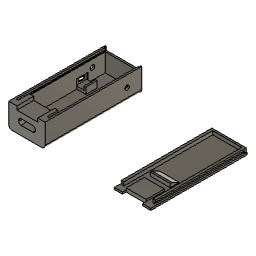
Coco_short_flat_Cover (Autodesk Fusion 360 design; units mm, degrees)
Autodesk Fusion 360 part; units mm, degrees
sketch "Skizze1" plane through (0, 0, 0) normal (0, 0, 1) x (1, 0, 0)
  line L0 (18, 20) -> (38, 20)
  line L1 (38, 20) -> (38, 73)
  line L2 (38, 73) -> (18, 73)
  line L3 (18, 73) -> (18, 20)
  line L4 (19, 23.2) -> (37, 23.2)
  line L5 (37, 23.2) -> (37, 72)
  line L6 (37, 72) -> (19, 72)
  line L7 (19, 72) -> (19, 23.2)
  line L8 (57, 90.4333) -> (57, 15.7858)
  line L9 (77, 72) -> (95, 72)
  line L10 (76, 73) -> (96, 73)
  line L11 (96, 73) -> (96, 20)
  line L12 (77, 23.2) -> (77, 72)
  line L13 (96, 20) -> (76, 20)
  line L14 (95, 72) -> (95, 23.2)
  line L15 (76, 20) -> (76, 73)
  line L16 (78, 71) -> (94, 71)
  line L17 (94, 71) -> (94, 23.2)
  line L18 (78, 23.2) -> (78, 71)
  line L19 (78, 71) -> (78, 73)
  line L20 (94, 71) -> (94, 73)
  line L21 (95, 72) -> (95, 73)
  line L22 (77, 72) -> (77, 73)
  line L23 (95, 23.2) -> (94, 23.2)
  line L24 (77, 23.2) -> (78, 23.2)
  line L25 (-15, -7.8) -> (-15, -6.8)
  line L26 (-15, -6.8) -> (-13, -6.8)
  line L27 (-13, -6.8) -> (-13, -15)
  line L28 (-13, -15) -> (-15, -15)
  line L29 (-15, -15) -> (-15, -14)
  line L30 (-15, -14) -> (-13.6, -14)
  line L31 (-13.6, -14) -> (-13.6, -7.8)
  line L32 (-13.6, -7.8) -> (-15, -7.8)
  dimension "d3" = 53
  dimension "d4" = 20
  dimension "d5" = 1
  dimension "d6" = 1
  dimension "d7" = 19
  dimension "d8" = 49.8
  dimension "d13" = 1
  dimension "d15" = 1
  dimension "d16" = 17
  dimension "d71" = 38
  dimension "d72" = 73
  dimension "d212" = 15
  dimension "d213" = 15
  dimension "d214" = 1
  dimension "d215" = 2
  dimension "d216" = 1.4
  dimension "d217" = 7.2
  dimension "d218" = 8.2
  dimension "d246" = 114
  constraint horizontal L0
  constraint vertical L1
  constraint horizontal L2
  constraint vertical L3
  constraint horizontal L4
  constraint vertical L5
  constraint horizontal L6
  constraint vertical L7
  constraint vertical L8
  constraint symmetric L0.start L8 L11.end
  constraint symmetric L0.end L8 L13.end
  constraint symmetric L1.end L8 L10.start
  constraint symmetric L2.end L8 L10.end
  constraint symmetric L4.start L8 L14.end
  constraint symmetric L4.end L8 L12.start
  constraint symmetric L5.end L8 L9.start
  constraint symmetric L6.end L8 L9.end
  constraint horizontal L16
  constraint vertical L17
  constraint vertical L18
  constraint coincident L10 L19.end
  constraint perpendicular L10 L19
  constraint coincident L10 L20.end
  constraint perpendicular L10 L20
  constraint coincident L10 L21.end
  constraint perpendicular L10 L21
  constraint coincident L10 L22.end
  constraint perpendicular L10 L22
  constraint perpendicular L14 L23
  constraint perpendicular L12 L24
  constraint vertical L25
  constraint perpendicular L25 L26
  constraint perpendicular L26 L27
  constraint perpendicular L27 L28
  constraint perpendicular L28 L29
  constraint perpendicular L27 L30
  constraint perpendicular L30 L31
  constraint perpendicular L25 L32
  constraint collinear L25 L29
  measures "d3" distance of L0 L2
  measures "d4" distance of L1 L3
  measures "d5" distance of L2 L6
  measures "d6" distance of L1 L5
  measures "d7" distance of L1 L7
  measures "d8" distance of L2 L4
  measures "d13" distance of L9 L16
  measures "d15" distance of L14 L17
  measures "d16" distance of L14 L18
  measures "d71" distance of origin L1
  measures "d72" distance of origin L2
  measures "d212" distance of origin L28
  measures "d213" distance of origin L29
  measures "d214" distance of L28 L30
  measures "d215" distance of L27 L29
  measures "d216" distance of L29 L31
  measures "d217" distance of L28 L32
  measures "d218" distance of L26 L28
extrude "Extrusion1" add sketch "Skizze1" along normal blind 13 contours L0 L1 L2 L3 makes body 1
extrude "Extrusion2" add sketch "Skizze1" along normal blind 1 contours L4 L5 L6 L7 bodies 1
extrude "Extrusion3" add sketch "Skizze1" along normal blind 3 separate body contours L9 L10 L19 L22 | L9 L12 L18 L19 L24 | L9 L10 L19 L20 | L9 L10 L20 L21 | L9 L14 L17 L20 L23 makes body 2
extrude "Extrusion4" add sketch "Skizze1" along normal blind 1 contours L9 L10 L19 L22 | L10 L11 L12 L13 L14 L15 L16 L17 L18 L21 L22 L23 L24 | L9 L10 L19 L20 | L9 L16 L19 L20 | L9 L10 L20 L21 bodies 2
fillet "Abrundung1" radius 2 2 edges at (38, 46.5, 0) (18, 46.5, 0) on bodies 1
ref_plane "Arbeitsebene1" through (28, 0, 0) normal (1, 0, 0) x (0, 1, 0)
sketch "Skizze2" plane through (28, 0, 0) normal (1, 0, 0) x (0, 1, 0)
  line L0 (23.2, 12) -> (73, 12)
  line L1 (73, 12) -> (73, 11)
  line L2 (73, 11) -> (23.2, 11)
  line L3 (23.2, 11) -> (23.2, 12)
  dimension "d25" = 11
  dimension "d26" = 49.8
  dimension "d27" = 1
  dimension "d44" = 73
  constraint horizontal L0
  constraint vertical L1
  constraint horizontal L2
  constraint vertical L3
  measures "d25" vertical distance of origin L2.end
  measures "d26" distance of L1 L3
  measures "d27" distance of L0 L2
  measures "d44" distance of origin L1
extrude "Extrusion10" cut sketch "Skizze2" along normal mid plane 19 bodies 1
sketch "Skizze3" plane through (0, 20, 0) normal (0, -1, 0) x (1, 0, 0)
  arc A0 (18, 2) -> (20, 0) centre (20, 2) ccw
  arc A1 (36, 0) -> (38, 2) centre (36, 2) ccw
  line L0 (38, 2) -> (38, 13)
  line L1 (38, 13) -> (18, 13)
  line L2 (18, 13) -> (18, 2)
  line L3 (24.69, 4.89) -> (31.31, 4.89)
  line L4 (24.69, 8.11) -> (31.31, 8.11)
  line L5 (28, 12.5188) -> (28, 0.4317)
  arc A2 (23.49, 6.09) -> (24.69, 4.89) centre (24.69, 6.09) ccw
  line L6 (23.49, 6.09) -> (23.49, 6.91)
  arc A3 (24.69, 8.11) -> (23.49, 6.91) centre (24.69, 6.91) ccw
  arc A4 (32.51, 6.91) -> (31.31, 8.11) centre (31.31, 6.91) ccw
  arc A5 (31.31, 4.89) -> (32.51, 6.09) centre (31.31, 6.09) ccw
  line L7 (32.51, 6.91) -> (32.51, 6.09)
  line L8 (22.5, 13) -> (34, 13)
  line L9 (34, 13) -> (34, 11)
  line L10 (34, 11) -> (22.5, 11)
  line L11 (22.5, 11) -> (22.5, 13)
  line L12 (20, 0) -> (36, 0)
  dimension "d30" = 6.62
  dimension "d32" = 6.62
  dimension "d34" = 3.31
  dimension "d35" = 3.31
  dimension "d36" = 1.2
  dimension "d37" = 1.2
  dimension "d171" = 2
  dimension "d204" = 6
  dimension "d205" = 11.5
  dimension "d269" = 4.89
  dimension "d270" = 8.11
  constraint horizontal L3
  constraint horizontal L4
  constraint tangent L3 A2
  constraint vertical L6
  constraint tangent L6 A3
  constraint tangent L4 A3
  constraint tangent A2 L6
  constraint tangent L4 A4
  constraint tangent L3 A5
  constraint perpendicular L1 L7
  constraint tangent A5 L7
  constraint tangent A4 L7
  constraint horizontal L8
  constraint vertical L9
  constraint horizontal L10
  constraint vertical L11
  constraint coincident L1 L8.start
  measures "d30" distance of L3.start L3.end
  measures "d32" distance of L4.start L4.end
  measures "d34" distance of L3.end L5
  measures "d35" distance of L4.end L5
  measures "d36" radius of A3
  measures "d37" radius of A4
  measures "d171" distance of L8 L10
  measures "d204" distance of L5 L9
  measures "d205" distance of L9 L11
  measures "d269" distance of origin L3
  measures "d270" distance of origin L4
extrude "Extrusion6" cut sketch "Skizze3" against normal blind 3.2 contours L1 L8 L9 L10 L11 | L3 L4 L5 A2 L6 A3 | L3 L4 L5 A4 A5 L7 bodies 1
fillet "Abrundung2" [suppressed]
sketch "Skizze7" plane through (0, 73, 0) normal (0, 1, 0) x (-1, 0, 0)
  arc A0 (-20, 0) -> (-18, 2) centre (-20, 2) ccw
  line L0 (-18, 2) -> (-18, 13)
  line L1 (-38, 13) -> (-38, 2)
  arc A1 (-38, 2) -> (-36, 0) centre (-36, 2) ccw
  line L2 (-36, 0) -> (-20, 0)
  line L3 (-37.5, 13) -> (-18.5, 13)
  line L4 (-18.5, 13) -> (-18.5, 12)
  line L5 (-18.5, 12) -> (-37.5, 12)
  line L6 (-37.5, 12) -> (-37.5, 13)
  line L7 (-28, 12.5188) -> (-28, 0.4317)
  circle A2 centre (-31.5, 6) radius 1.25
  line L8 (-18, 13) -> (-38, 13)
  line L9 (-18.5, 12) -> (-18.5, 11)
  line L10 (-18.5, 11) -> (-37.5, 11)
  line L11 (-37.5, 11) -> (-37.5, 12)
  line L12 (-37.5, 12) -> (-18.5, 12)
  dimension "d59" = 19
  dimension "d60" = 9.5
  dimension "d116" = 2.5
  dimension "d117" = 6
  dimension "d206" = 3.5
  dimension "d264" = 13
  dimension "d265" = 1
  constraint horizontal L3
  constraint vertical L4
  constraint horizontal L5
  constraint vertical L6
  measures "d59" distance of L4 L6
  measures "d60" distance of L4 L7
  measures "d116" diameter of A2
  measures "d117" distance of L2 A2.centre
  measures "d206" distance of L7 A2.centre
  measures "d264" distance of origin L3
  measures "d265" distance of L3 L5
extrude "Extrusion11" cut sketch "Skizze7" against normal blind 1 contours L3 L4 L5 L6 L8 L12 bodies 1
sketch "Skizze8" plane through (95, 0, 0) normal (1, 0, 0) x (0, 1, 0)
  line L0 (23.2, 1) -> (73, 1)
  line L1 (73, 1) -> (73, 3)
  line L2 (73, 3) -> (23.2, 3)
  line L3 (23.2, 3) -> (73, 3)
  line L4 (72, 2.1) -> (23.2, 2.1)
  line L5 (23.2, 2.1) -> (23.2, 3)
  line L6 (73, 3) -> (73, 1)
  line L7 (72, 1) -> (72, 2.1)
  line L8 (23.2, 3) -> (23.2, 1)
  dimension "d63" = 0.9
  dimension "d125" = 1
  constraint horizontal L3
  constraint horizontal L4
  constraint vertical L5
  constraint coincident L2.end L3.start
  constraint coincident L0.end L1.start
  constraint coincident L0 L7.start
  constraint coincident L4 L7.end
  constraint perpendicular L4 L7
  constraint coincident L1.end L2.start
  measures "d63" distance of L2.end L4.end
  measures "d125" distance of L6 L7
extrude "Extrusion12" add sketch "Skizze8" along normal blind 0.4 contours L0 L1 L2 L3 L4 L5 L6 L7 L8 bodies 2
sketch "Skizze9" plane through (77, 0, 0) normal (-1, 0, 0) x (0, -1, 0)
  line L0 (-23.2, 3) -> (-23.2, 2.1)
  line L1 (-23.2, 2.1) -> (-72, 2.1)
  line L2 (-73, 1) -> (-73, 3)
  line L3 (-73, 1) -> (-72, 1)
  line L4 (-72, 2.1) -> (-72, 1)
  line L5 (-23.2, 1) -> (-23.2, 3)
  line L6 (-73, 1) -> (-23.2, 1)
  line L7 (-73, 3) -> (-23.2, 3)
  line L8 (-73, 1) -> (-73, 3)
  line L9 (-23.2, 1) -> (-23.2, 3)
  dimension "d127" = 1
  dimension "d268" = 0.9
  constraint vertical L0
  constraint horizontal L1
  constraint vertical L2
  constraint coincident L1 L4.start
  constraint coincident L1.end L4
  constraint coincident L0.start L5.end
  constraint collinear L2 L8
  constraint collinear L3 L6
  measures "d127" distance of L2 L4
  measures "d268" distance of L1 L7
extrude "Extrusion13" add sketch "Skizze9" along normal blind 0.4 contours L0 L1 L2 L3 L4 L5 L6 L7 L8 L9 bodies 2
sketch "Skizze10" plane through (0, 0, 1) normal (0, 0, 1) x (-1, 0, 0)
  line L0 (-76, -20) -> (-96, -20)
  line L1 (-94, -23.2) -> (-94, -72)
  line L2 (-80.5, -32) -> (-91.5, -32)
  line L3 (-80.5, -32) -> (-80.5, -22)
  line L4 (-80.5, -22) -> (-91.5, -22)
  line L5 (-91.5, -22) -> (-91.5, -32)
  line L6 (-80.5, -40.2) -> (-91.5, -40.2)
  line L7 (-91.5, -40.2) -> (-91.5, -35.2)
  line L8 (-91.5, -35.2) -> (-80.5, -35.2)
  line L9 (-80.5, -35.2) -> (-80.5, -40.2)
  line L10 (-95.4, -72) -> (-95, -72)
  line L11 (-95, -72) -> (-95, -23.2)
  line L12 (-95, -23.2) -> (-94, -23.2)
  line L13 (-76.6, -73) -> (-76, -73)
  line L14 (-76, -73) -> (-76, -20)
  line L15 (-96, -20) -> (-96, -73)
  line L16 (-96, -73) -> (-95.4, -73)
  line L17 (-95.4, -73) -> (-95.4, -72)
  line L18 (-76.6, -72) -> (-76.6, -73)
  line L19 (-76.6, -73) -> (-95.4, -73)
  line L20 (-94, -72) -> (-78, -72)
  line L21 (-78, -72) -> (-78, -23.2)
  line L22 (-78, -23.2) -> (-77, -23.2)
  line L23 (-77, -23.2) -> (-77, -72)
  dimension "d226" = 2
  dimension "d227" = 12
  dimension "d249" = 20.2
  dimension "d250" = 15.2
  dimension "d271" = 15.5
  dimension "d272" = 4.5
  constraint perpendicular L2 L3
  constraint perpendicular L2 L5
  constraint horizontal L6
  constraint vertical L7
  constraint horizontal L8
  constraint vertical L9
  constraint collinear L3 L9
  constraint collinear L5 L7
  measures "d226" distance of L0 L4
  measures "d227" distance of L0 L2
  measures "d249" distance of L0 L6
  measures "d250" distance of L0 L8
  measures "d271" distance of L5 L14
  measures "d272" distance of L3 L14
extrude "Extrusion30" add sketch "Skizze10" along normal blind 1 contours L2 L3 L4 L5 bodies 2
extrude "Extrusion33" add sketch "Skizze10" along normal blind 2 contours L6 L7 L8 L9 bodies 2
chamfer "Fase2" distance 4 distance2 2 1 edges at (86, 40.2, 3) measured on face at (84.1667, 38.5333, 3) on bodies 2
sketch "Skizze11" plane through (18, 0, 0) normal (-1, 0, 0) x (0, -1, 0)
  line L0 (-73, 2) -> (-20, 2)
  line L1 (-20, 2) -> (-20, 13)
  line L2 (-20, 13) -> (-73, 13)
  line L3 (-73, 13) -> (-73, 2)
  line L4 (-61.2, 3.4) -> (-57.9, 3.4)
  line L5 (-57.9, 3.4) -> (-57.9, 5)
  line L6 (-57.9, 5) -> (-61.2, 5)
  line L7 (-61.2, 5) -> (-61.2, 3.4)
  line L8 (-56.5, 5.95) -> (-56.5, 2.45)
  line L9 (-56.5, 5.95) -> (-62.6, 5.95)
  line L10 (-62.6, 5.95) -> (-62.6, 2.45)
  line L11 (-62.6, 2.45) -> (-56.5, 2.45)
  circle A0 centre (-65, 7) radius 1.25
  dimension "d76" = 3.3
  dimension "d77" = 1.6
  dimension "d78" = 15.1
  dimension "d179" = 3.95
  dimension "d180" = 3.5
  dimension "d181" = 16.5
  dimension "d182" = 6.1
  dimension "d193" = 3
  dimension "d258" = 6
  dimension "d259" = 8
  dimension "d260" = 2.5
  constraint horizontal L4
  constraint vertical L5
  constraint horizontal L6
  constraint vertical L7
  constraint perpendicular L6 L8
  constraint perpendicular L8 L9
  constraint perpendicular L0 L10
  constraint horizontal L11
  measures "d76" distance of L4.start L4.end
  measures "d77" distance of L4.start L6.end
  measures "d78" distance of L3 L5
  measures "d179" distance of L0 L9
  measures "d180" distance of L9 L11
  measures "d181" distance of L3 L8
  measures "d182" distance of L8 L10
  measures "d193" distance of L0 L6
  measures "d258" distance of L2 A0.centre
  measures "d259" distance of L3 A0.centre
  measures "d260" diameter of A0
extrude "Extrusion15" cut sketch "Skizze11" against normal blind 1 contours L4 L5 L6 L7 bodies 1
extrude "Extrusion34" cut sketch "Skizze11" against normal blind 20 contours A0 bodies 1
sketch "Skizze12" plane through (0, 0, 1) normal (0, 0, 1) x (-1, 0, 0)
  line L0 (-19, -72) -> (-19, -23.2)
  line L1 (-37, -23.2) -> (-37, -72)
  line L2 (-23, -62.5) -> (-23, -56.4)
  line L3 (-24, -62.5) -> (-24, -56.4)
  line L4 (-24, -56.4) -> (-23, -56.4)
  line L5 (-24, -62.5) -> (-23, -62.5)
  line L6 (-18, -73) -> (-18, -20)
  line L7 (-23, -62.5) -> (-19, -62.5)
  line L8 (-23, -56.4) -> (-19, -56.4)
  line L9 (-18.5, -73) -> (-18, -73)
  line L10 (-19, -23.2) -> (-37, -23.2)
  line L11 (-34, -20) -> (-38, -20)
  line L12 (-18, -20) -> (-22.5, -20)
  dimension "d177" = 6
  dimension "d178" = 5
  dimension "d253" = 10.5
  dimension "d254" = 16.6
  constraint vertical L2
  constraint perpendicular L3 L4
  constraint vertical L3
  constraint perpendicular L2 L5
  constraint coincident L0 L7.end
  constraint perpendicular L0 L7
  constraint coincident L0 L8.end
  constraint perpendicular L0 L8
  measures "d177" distance of L3 L6
  measures "d178" distance of L2 L6
  measures "d253" distance of L7 L9
  measures "d254" distance of L8 L9
extrude "Extrusion17" add sketch "Skizze12" along normal blind 3.5 contours L2 L3 L4 L5 bodies 1
extrude "Extrusion27" add sketch "Skizze12" along normal blind 1.45 contours L0 L2 L7 L8 bodies 1
sketch "Skizze13" plane through (19, 0, 0) normal (1, 0, 0) x (0, 1, 0)
  line L0 (72, 1) -> (72, 11)
  line L1 (62.5, 1) -> (72, 1)
  line L2 (61.2, 3.4) -> (57.9, 3.4)
  line L3 (57.9, 3.4) -> (57.9, 5)
  line L4 (57.9, 5) -> (61.2, 5)
  line L5 (61.2, 5) -> (61.2, 3.4)
  line L6 (-70.5, 1.05) -> (-64.4, 1.05)
  line L7 (-64.4, 4.55) -> (-64.4, 1.05)
  line L8 (-65.9, 2) -> (-65.9, 3.6)
  line L9 (-69, 2) -> (-65.9, 2)
  line L10 (-64.4, 4.55) -> (-70.5, 4.55)
  line L11 (-70.5, 4.55) -> (-70.5, 1.05)
  line L12 (-69, 3.6) -> (-69, 2)
  line L13 (-65.9, 3.6) -> (-69, 3.6)
  line L14 (56.4, 5.95) -> (56.4, 1)
  line L15 (62.5, 1) -> (62.5, 5.95)
  line L16 (62.5, 5.95) -> (56.4, 5.95)
  line L17 (73, 13) -> (73, 2)
  line L18 (62.6, 2.45) -> (56.5, 2.45)
  line L19 (62.5, 2.45) -> (62.5, 1)
  line L20 (56.4, 1) -> (56.4, 2.45)
  line L21 (56.4, 2.45) -> (62.5, 2.45)
  circle A0 centre (65, 7) radius 1.25
  line L22 (23.2, 11) -> (23.2, 1)
  line L23 (72, 11) -> (23.2, 11)
  line L24 (23.2, 1) -> (56.4, 1)
  point P0 (-83, 2)
  dimension "d183" = 3.1
  dimension "d184" = 1.6
  dimension "d185" = 3.5
  dimension "d186" = 6.1
  dimension "d187" = 6.1
  dimension "d188" = 16.6
  dimension "d189" = 3.5
  constraint horizontal L9
  constraint vertical L8
  constraint horizontal L13
  constraint vertical L12
  constraint perpendicular L7 L13
  constraint perpendicular L7 L10
  constraint horizontal L6
  constraint coincident L1 L14.end
  constraint perpendicular L1 L14
  constraint coincident L1 L15.start
  constraint perpendicular L1 L15
  constraint perpendicular L14 L16
  measures "d183" distance of L9.start L8.start
  measures "d184" distance of L9.start L12.start
  measures "d185" distance of L6 L10
  measures "d186" distance of L7 L11
  measures "d187" distance of L14 L15
  measures "d188" distance of L14 L17
  measures "d189" distance of L16 L18
extrude "Extrusion26" cut sketch "Skizze13" against normal blind 0.5 contours L14 L15 L16 L18 L21 bodies 1
sketch "Skizze14" plane through (0, 20, 0) normal (0, -1, 0) x (1, 0, 0)
  line L0 (76, 0) -> (96, 0)
  line L1 (80.5, 1) -> (91.5, 1)
  line L2 (91.5, 1) -> (91.5, 0)
  line L3 (91.5, 0) -> (80.5, 0)
  line L4 (80.5, 0) -> (80.5, 1)
  line L5 (96, 0) -> (96, 1)
  line L6 (76, 1) -> (76, 0)
  line L7 (96, 1) -> (76, 1)
  dimension "d106" = 11
  dimension "d267" = 15.5
  constraint horizontal L1
  constraint vertical L2
  constraint horizontal L3
  constraint vertical L4
  constraint collinear L0 L3
  constraint collinear L1 L7
  measures "d106" distance of L2 L4
  measures "d267" distance of L2 L6
extrude "Extrusion20" cut sketch "Skizze14" against normal blind 2 contours L0 L1 L2 L3 L4 L7 bodies 2
ref_plane "Arbeitsebene2" through (0, 0, 6) normal (0, 0, 1) x (1, 0, 0)
sketch "Skizze15" plane through (0, 0, 6) normal (0, 0, 1) x (1, 0, 0)
  line L0 (24, 73) -> (24, 76)
  arc A0 (27, 79) -> (24, 76) centre (27, 76) ccw
  arc A1 (34, 76) -> (31, 79) centre (31, 76) ccw
  line L1 (27, 79) -> (31, 79)
  line L2 (34, 76) -> (34, 73)
  line L3 (18, 73) -> (18, 20)
  line L4 (18.5, 73) -> (18, 73)
  dimension "d112" = 16
  dimension "d113" = 10
  dimension "d114" = 3
  dimension "d115" = 3
  dimension "d255" = 3
  constraint vertical L0
  constraint tangent L0 A0
  constraint tangent A0 L1
  constraint perpendicular L1 L2
  constraint tangent A1 L1
  constraint tangent A1 L2
  constraint vertical L2
  measures "d112" distance of L2 L3
  measures "d113" distance of L0 L2
  measures "d114" radius of A0
  measures "d115" radius of A1
  measures "d255" distance of A0.centre L4
sweep "Sweeping1" [suppressed]
fillet "Abrundung5" [suppressed]
sketch "Skizze16" plane through (0, 0, 0) normal (0, 0, -1) x (1, 0, 0)
  line L0 (20, -20) -> (20, -73)
  line L1 (20, -73) -> (36, -73)
  line L2 (36, -73) -> (36, -20)
  circle A0 centre (28, -28) radius 7
  circle A1 centre (28, -28) radius 6
  line L3 (38, -73) -> (38, -20)
  circle A2 centre (28, -28) radius 3
  circle A3 centre (28, -28) radius 1.5
  line L4 (22.9049, -23.2) -> (33.0951, -23.2)
  line L5 (36, -20) -> (20, -20)
  dimension "d128" = 14
  dimension "d130" = 10
  dimension "d131" = 1
  dimension "d132" = 6
  dimension "d133" = 3
  dimension "d273" = 8
  dimension "d274" = 3.2
  constraint concentric A0 A1
  constraint concentric A0 A2
  constraint concentric A1 A3
  constraint coincident A0 L4.start
  constraint coincident A0 L4.end
  constraint horizontal L4
  measures "d128" diameter of A0
  measures "d130" distance of A0.centre L3
  measures "d131" distance of A0 A1
  measures "d132" diameter of A2
  measures "d133" diameter of A3
  measures "d273" distance of A0.centre L5
  measures "d274" distance of L4 L5
extrude "Extrusion32" cut sketch "Skizze16" against normal blind 1 contours A0 A1 L4 | A2 | A3 picked at (23.4498, -32.8545) bodies 1
extrude "Extrusion22" add sketch "Skizze16" against normal blind 1 separate body contours A0 A1 L4 | A2 | A3 picked at (23.4498, -32.8545) makes body 3 at (27.9253, 27.1355, 0) makes body 4 at (25.6704, 34.601, 0.6667)
sketch "Skizze17" plane through (0, 23.2, 0) normal (0, 1, 0) x (-1, 0, 0)
  line L0 (-20.1, 13) -> (-20.1, 12)
  line L1 (-35.9, 12) -> (-35.9, 13)
  line L2 (-37, 12) -> (-37, 13)
  line L3 (-34, 13) -> (-37, 13)
  line L4 (-38, 2) -> (-38, 13)
  line L5 (-34, 11) -> (-22.5, 11)
  line L6 (-35, 10) -> (-35, 12)
  line L7 (-35.9, 12) -> (-35, 12)
  line L8 (-21.5, 12) -> (-20.1, 12)
  line L9 (-20.1, 13) -> (-22.5, 13)
  line L10 (-21.5, 12) -> (-21.5, 10)
  line L11 (-35.9, 13) -> (-34, 13)
  line L12 (-37, 12) -> (-37.5, 12)
  line L13 (-35, 10) -> (-21.5, 10)
  line L14 (-22.5, 11) -> (-22.5, 13)
  line L15 (-22.5, 13) -> (-22.5, 11)
  line L16 (-34, 11) -> (-34, 13)
  line L17 (-37, 13) -> (-37, 12)
  line L18 (-19, 1) -> (-19, 11)
  line L19 (-34, 13) -> (-34, 11)
  line L20 (-37.5, 12) -> (-37.5, 11)
  line L21 (-37.5, 11) -> (-37, 11)
  line L22 (-37, 11) -> (-37, 1)
  line L23 (-37, 1) -> (-33.0951, 1)
  line L24 (-33.0951, 1) -> (-33.0951, 0)
  line L25 (-33.0951, 0) -> (-31.6, 0)
  line L26 (-31.6, 0) -> (-31.6, 1)
  line L27 (-31.6, 1) -> (-24.4, 1)
  line L28 (-24.4, 1) -> (-24.4, 0)
  line L29 (-24.4, 0) -> (-22.9049, 0)
  line L30 (-22.9049, 0) -> (-22.9049, 1)
  line L31 (-22.9049, 1) -> (-19, 1)
  line L32 (-19, 11) -> (-18.5, 11)
  line L33 (-18.5, 11) -> (-18.5, 12)
  line L34 (-18.5, 12) -> (-19, 12)
  line L35 (-19, 12) -> (-19, 13)
  line L36 (-19, 13) -> (-22.5, 13)
  line L37 (-23.49, 6.91) -> (-23.49, 6.09)
  arc A0 (-24.69, 4.89) -> (-23.49, 6.09) centre (-24.69, 6.09) ccw
  line L38 (-24.69, 4.89) -> (-31.31, 4.89)
  arc A1 (-32.51, 6.09) -> (-31.31, 4.89) centre (-31.31, 6.09) ccw
  line L39 (-32.51, 6.09) -> (-32.51, 6.91)
  arc A2 (-31.31, 8.11) -> (-32.51, 6.91) centre (-31.31, 6.91) ccw
  line L40 (-31.31, 8.11) -> (-24.69, 8.11)
  arc A3 (-23.49, 6.91) -> (-24.69, 8.11) centre (-24.69, 6.91) ccw
  line L41 (-18.5, 12) -> (-19, 12)
  line L42 (-37, 12) -> (-37.5, 12)
  line L43 (-37, 13) -> (-34, 13)
  dimension "d174" = 2.1
  dimension "d175" = 17.9
  dimension "d266" = 1
  dimension "d275" = 3
  dimension "d277" = 1
  dimension "d278" = 2
  dimension "d279" = 1
  constraint vertical L0
  constraint vertical L1
  constraint perpendicular L6 L7
  constraint vertical L6
  constraint perpendicular L0 L8
  constraint coincident L3.start L11.end
  constraint collinear L7 L8
  constraint perpendicular L10 L13
  constraint perpendicular L9 L14
  constraint collinear L14 L15
  constraint horizontal L5
  constraint vertical L19
  measures "d174" distance of L1 L4
  measures "d175" distance of L0 L4
  measures "d266" distance of L7 L11
  measures "d275" distance of L11 L13
  measures "d277" distance of L6 L16
  measures "d278" distance of L5 L11
  measures "d279" distance of L10 L14
extrude "Extrusion25" add sketch "Skizze17" along normal blind 6 contours L0 L1 L3 L5 L6 L7 L8 L9 L10 L11 L13 L14 L15 L16 L19 L36 L43 bodies 1
extrude "Extrusion28" add sketch "Skizze1" along normal blind 4 separate body contours L25 L26 L27 L28 L29 L30 L31 L32 makes body 5
sketch "Skizze18" plane through (-13.6, 0, 0) normal (-1, 0, 0) x (0, -1, 0)
  line L0 (7.8, 0) -> (14, 0)
  line L1 (14, 0) -> (14, 4)
  line L2 (14, 4) -> (7.8, 4)
  line L3 (7.8, 4) -> (7.8, 0)
  line L4 (7.8, 0) -> (14, 0)
  line L5 (14, 0) -> (14, 1.5)
  line L6 (14, 1.5) -> (7.8, 1.5)
  line L7 (7.8, 1.5) -> (7.8, 0)
  dimension "d221" = 1.5
  constraint horizontal L4
  constraint vertical L5
  constraint horizontal L6
  constraint vertical L7
  constraint coincident L1 L5.end
  constraint coincident L0.start L3.end
  measures "d221" distance of L4 L6
extrude "Extrusion29" cut sketch "Skizze18" against normal blind 0.6 contours L0 L1 L3 L4 L5 L6 L7 bodies 5
sketch "Skizze19" plane through (0, 0, 6) normal (0, 0, 1) x (1, 0, 0)
  circle A0 centre (29, 80) radius 10
  line L0 (18, 73) -> (18, 20)
  line L1 (14, 95) -> (44, 95)
  line L2 (44, 95) -> (44, 73)
  line L3 (14, 73) -> (14, 95)
  line L4 (18.5, 73) -> (18, 73)
  line L5 (44, 73) -> (14, 73)
  dimension "d231" = 20
  dimension "d233" = 11
  dimension "d234" = 15
  dimension "d235" = 30
  dimension "d236" = 15
  dimension "d256" = 7
  dimension "d257" = 7
  constraint horizontal L1
  constraint vertical L2
  constraint vertical L3
  constraint perpendicular L3 L5
  measures "d231" diameter of A0
  measures "d233" distance of A0.centre L0
  measures "d234" distance of A0.centre L2
  measures "d235" distance of L2 L3
  measures "d236" distance of A0.centre L1
  measures "d256" distance of A0.centre L4
  measures "d257" distance of A0.centre L5
hidden bodies 3 4 5
equation "d3 = Länge + Wandstärke"
equation "d4 = Breite + 2 * Wandstärke"
equation "d5 = Wandstärke"
equation "d6 = Wandstärke"
equation "d7 = Breite + Wandstärke"
equation "d8 = d3 - 3.2 mm"
equation "d9 = Höhe_Gehäuse"
equation "d11 = Wandstärke"
equation "d16 = Breite - 1 mm"
equation "d17 = Höhe_Deckel + 2 mm"
equation "d19 = Höhe_Deckel"
equation "d23 = Breite + 20 mm - Breite / 2 - Wandstärke"
equation "d25 = Höhe_Gehäuse - 2 mm"
equation "d26 = Länge + Wandstärke - 3.2 mm"
equation "d30 = d34 * 2"
equation "d32 = d30"
equation "d35 = d34"
equation "d44 = Länge + Wandstärke + 20 mm"
equation "d56 = Höhe_Deckel"
equation "d57 = Breite / 2 + 0.5 mm"
equation "d59 = Breite + 1 mm"
equation "d60 = Breite / 2 + 0.5 mm"
equation "d71 = Breite + 20 mm"
equation "d72 = Länge + 21 mm"
equation "d79 = -Wandstärke"
equation "d130 = Breite / 2 + Wandstärke"
equation "d175 = Breite + Wandstärke - 1.1 mm"
equation "d178 = d177 - 1 mm"
equation "d179 = d193 - d77 / 2 + d180 / 2"
equation "d181 = d78 + d182 / 2 - d76 / 2"
equation "Länge = 52 mm"
equation "Breite = 18 mm"
equation "Wandstärke = 1 mm"
equation "Höhe_Gehäuse = 13 mm"
equation "Höhe_Deckel = 1 mm"
equation "d216 = d215 - 0.6 mm"
equation "d217 = d218 - 1 mm"
equation "d234 = d231 / 2 + 5 mm"
equation "d235 = d234 * 2"
equation "d236 = d231 / 2 + 5 mm"
equation "d246 = d71 * 3"
equation "d249 = d250 + 5 mm"
equation "d253 = Wandstärke + 9.5 mm"
equation "d254 = Wandstärke + 15.6 mm"
equation "d258 = Höhe_Gehäuse / 2 - 0.5 mm"
equation "d261 = -Breite - 2 * Wandstärke"
equation "d264 = Höhe_Gehäuse"
equation "d267 = Breite / 4 + 11 mm"
equation "d271 = d272 + 11 mm"
equation "d272 = Breite / 4"
named bodies: "Gehäuse", "Deckel"
